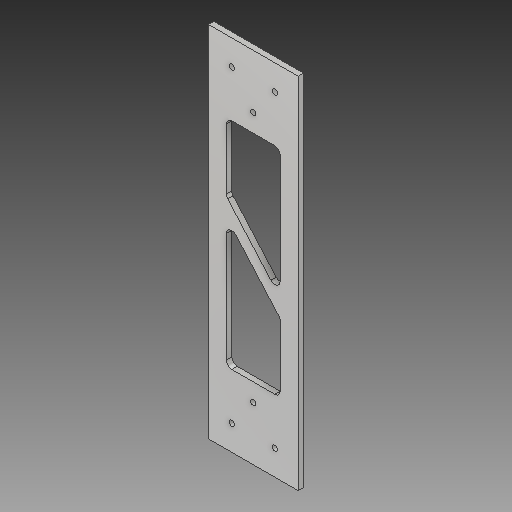
# Autodesk Inventor part: Bok
Saved by Autodesk Inventor 2018 (Build 220112000, 112)
## iProperties
Created: 2018-08-13
Part Number: Bok
Material: Aluminium 6061
Document SubType Name: Modeling
Designer: Wojciech
Density: 2.7 g/cm^3
Appearance: Aluminium — ciemne
Mass: 54.2008 g
Surface Area: 160.969 cm^2
Volume: 20.0744 cm^3
Author: Wojciech
Autodesk Inventor part; units mm, degrees
ref_plane "YZ Plane" through (0, 0, 0) normal (1, 0, 0) x (0, 1, 0)
ref_plane "XZ Plane" through (0, 0, 0) normal (0, 1, 0) x (-1, 0, 0)
ref_plane "XY Plane" through (0, 0, 0) normal (0, 0, 1) x (1, 0, 0)
sketch "Szkic1" plane through (0, 0, 0) normal (0, 0, 1) x (1, 0, 0)
  line L0 (-25, -100) -> (25, -100)
  line L1 (25, -100) -> (25, 100)
  line L2 (25, 100) -> (-25, 100)
  line L3 (-25, 100) -> (-25, -100)
  line L4 (-25, -100) -> (25, 100) construction
  line L5 (25, -100) -> (-25, 100) construction
  point P0 (0, 0)
  dimension "d0" = 50
  dimension "d1" = 200
  constraints: 12 end point, 2 midpoint, 2 parallel, 1 horizontal, 1 perpendicular
  measures "d0" distance of L2.end L1.end
  measures "d1" distance of L1.end L0.end
extrude "Wyciągnięcie proste1" add sketch "Szkic1" along normal blind 3
sketch "Szkic3" plane through (0, 0, 3) normal (0, 0, 1) x (1, 0, 0)
  line L0 (-25, -100) -> (25, -100) projected
  line L1 (25, 100) -> (-25, 100) projected
  line L2 (0, 100) -> (0, -100) construction
  line L3 (-25, 100) -> (-25, -100) projected
  line L4 (-25, 0) -> (25, 0) construction
  point P0 (0, 0)
  point P1 (-12, -86)
  point P2 (12, -86)
  point P3 (0, -70)
  point P4 (-12, 86)
  point P5 (12, 86)
  point P6 (0, 70)
  dimension "d21" = 14
  dimension "d22" = 14
  dimension "d23" = 24
  dimension "d24" = 12
  dimension "d25" = 30
  constraints: 4 end point, 3 midpoint, 3 symmetric about line, 1 horizontal, 1 point on line
  measures "d21" distance from line of L0 point (-12, -86)
  measures "d22" distance from line of L0 point (12, -86)
  measures "d23" distance of point (12, -86) point (-12, -86)
  measures "d24" distance from line of point (-12, -86) L2
  measures "d25" distance from line of L0 point (0, -70)
hole "Otwór1" at (-12, -86, 3) at (12, -86, 3) at (0, -70, 3) at (0, 70, 3) at (12, 86, 3) at (-12, 86, 3) direction (0, 0, -1) diameter 3 depth 8 tip angle 118
sketch "Szkic4" plane through (0, 0, 3) normal (0, 0, 1) x (1, 0, 0)
  line L0 (-25, 100) -> (-25, -100) projected
  line L1 (25, -100) -> (25, 100) projected
  line L2 (15, -12) -> (0, 5)
  line L3 (-15, 60) -> (-15, 22)
  line L4 (0, 5) -> (-15, 22)
  line L5 (-15, 60) -> (15, 60)
  line L6 (25, -100) -> (25, 100) projected
  line L7 (15, 60) -> (15, -12)
  line L8 (-15, -60) -> (15, -60)
  line L9 (15, -60) -> (15, -22)
  line L10 (15, -22) -> (-15, 12)
  line L11 (-15, 12) -> (-15, -60)
  point P0 (0, 0)
  dimension "d33" = 10
  dimension "d34" = 10
  dimension "d35" = 60
  dimension "d36" = 60
  dimension "d37" = 5
  dimension "d38" = 25
  dimension "d39" = 10
  dimension "d40" = 12
  dimension "d41" = 10
  dimension "d42" = 10
  dimension "d43" = 10
  dimension "d44" = 10
  dimension "d45" = 60
  dimension "d46" = 60
  constraints: 18 end point, 1 coincident, 1 collinear, 1 parallel, 1 perpendicular, 1 vertical
  measures "d33" distance from line of L0 L3.start
  measures "d34" distance from line of L1 L5.end
  measures "d35" vertical distance of L3.start point (0, 0)
  measures "d36" vertical distance of point (0, 0) L5.end
  measures "d37" distance of point (0, 0) L2.end
  measures "d38" distance from line of L0 L2.end
  measures "d39" distance from line of L1 L2.start
  measures "d40" vertical distance of point (0, 0) L2.start
  measures "d41" distance of L10.end L3.end
  measures "d42" distance of L9.end L2.start
  measures "d43" distance from line of L1 L9.end
  measures "d44" distance from line of L0 L10.end
  measures "d45" vertical distance of L8.end point (0, 0)
  measures "d46" vertical distance of L8.start point (0, 0)
extrude "Wyciągnięcie proste3" cut sketch "Szkic4" against normal blind 3
fillet "Zaokrąglenie1" radius 3 8 edges at (15, -12, 1.5) (-15, 22, 1.5) (15, 60, 1.5) (-15, 60, 1.5) (-15, 12, 1.5) (15, -22, 1.5) (-15, -60, 1.5) (15, -60, 1.5)
